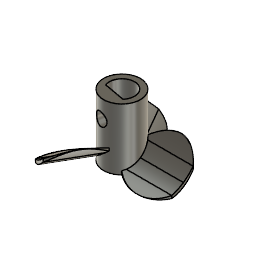
Drill_head_ship_screw (Autodesk Fusion 360 design; units mm, degrees)
Autodesk Fusion 360 part; units mm, degrees
note: some values were not read from the file. Chosen so that the rebuilt part matches the saved one: a direction; which face or edge a step refers to. Set by a fixed rule: which sketch regions a step uses.
sketch "Skizze1" plane through (0, 0, 0) normal (0, 0, 1) x (1, 0, 0)
  circle A0 centre (0, 0) radius 20
  dimension "d1" = 40
  constraint coincident A0.centre origin
  measures "d1" diameter of A0
extrude "Extrusion1" add sketch "Skizze1" along normal blind 10 makes body 1
sketch "Skizze2" plane through (0, 0, 10) normal (0, 0, 1) x (-1, 0, 0)
  circle A0 centre (0, 0) radius 20
  spline S0 degree 5 poles (-19.6944, -3.4827) (-19.4886, -3.7223) (-19.0692, -4.1829) (-18.4174, -4.8178) (-17.5023, -5.5517) (-16.2812, -6.2762) (-14.9841, -6.8018) (-13.6162, -7.1226) (-12.1897, -7.2366) (-10.7248, -7.1467) (-9.2455, -6.859) (-7.7765, -6.381) (-6.3398, -5.7215) (-4.9513, -4.8904) (-3.6191, -3.8981) (-2.3472, -2.7537) (-1.3783, -1.7223) (-0.6787, -0.8855) (-0.2242, -0.2998) (0, 0) knots 0 0 0 0 0 0 0.066667 0.133333 0.2 0.266667 0.333333 0.4 0.466667 0.533333 0.6 0.666667 0.733333 0.8 0.866667 0.933333 1 1 1 1 1 1
  line L0 (0, 0) -> (-20, 0) construction
  spline S1 degree 5 poles (-19.6944, 3.4827) (-19.4886, 3.7223) (-19.0692, 4.1829) (-18.4174, 4.8178) (-17.5023, 5.5517) (-16.2812, 6.2762) (-14.9841, 6.8018) (-13.6162, 7.1226) (-12.1897, 7.2366) (-10.7248, 7.1467) (-9.2455, 6.859) (-7.7765, 6.381) (-6.3398, 5.7215) (-4.9513, 4.8904) (-3.6191, 3.8981) (-2.3472, 2.7537) (-1.3783, 1.7223) (-0.6787, 0.8855) (-0.2242, 0.2998) (0, 0) knots 0 0 0 0 0 0 0.066667 0.133333 0.2 0.266667 0.333333 0.4 0.466667 0.533333 0.6 0.666667 0.733333 0.8 0.866667 0.933333 1 1 1 1 1 1
  line L1 (-21.3276, -1.5819) -> (-18.0612, -5.3835)
  line L2 (-1.5119, -2.0215) -> (1.5119, 2.0215)
  line L3 (-21.3276, 1.5819) -> (-18.0612, 5.3835)
  line L4 (-1.5119, 2.0215) -> (1.5119, -2.0215)
  point P0 (-14, -7)
  point P1 (-7, -6)
  point P2 (-14, 7)
  point P3 (-7, 6)
  constraint coincident A0 S0.start
  constraint coincident A0.centre S0.end
  constraint coincident A0 L0.end
  constraint horizontal L0
  constraint midpoint S0.start L1
  constraint midpoint A0.centre L2
  constraint symmetric S0.start L0 S1.start
  constraint symmetric P0 L0 P2
  constraint symmetric P1 L0 P3
  constraint symmetric A0.centre L0 S0.end
  constraint symmetric L0 L1.start L3.start
  constraint symmetric L0 L1.end L3.end
  constraint symmetric L0 L2.start L4.start
  constraint symmetric L0 L2.end L4.end
extrude "Extrusion2" cut sketch "Skizze2" against normal blind 38 contours A0 S0 S1 picked at (11.5447, -6.597) bodies 1
ref_plane "Arbeitsebene1" through (20, 0, 7.0602) normal (1, 0, 0) x (0, -1, 0)
sketch "Skizze3" plane through (20, 0, 0) normal (1, 0, 0) x (0, 1, 0)
  line L0 (0, 0) -> (-7.1861, 0)
  line L1 (-3.4827, 0) -> (-3.4827, 10)
  line L2 (0, 10) -> (-7.186, 10)
  line L3 (0, 10) -> (0, 0)
  line L4 (0, 0) -> (7.186, 0)
  line L5 (0, 0) -> (0, 10)
  line L6 (0, 10) -> (7.186, 10)
  line L7 (3.4827, 10) -> (3.4827, 0)
  line L8 (-3.4827, 10) -> (-3.4827, 0)
  line L9 (3.4827, 0) -> (-3.4827, 0)
  line L10 (3.4827, 0) -> (3.4827, 10)
  line L11 (3.4827, 10) -> (-3.4827, 10)
  spline S0 degree 5 poles (-7.1861, 0) (-6.8583, 0.0244) (-6.2065, 0.089) (-5.2397, 0.2335) (-3.9728, 0.523) (-2.4286, 1.0564) (-0.9268, 1.7751) (0.5297, 2.691) (1.9406, 3.8055) (3.309, 5.1055) (4.6386, 6.5747) (5.674, 7.8733) (6.4357, 8.9119) (6.937, 9.6326) (7.186, 10) knots 0 0 0 0 0 0 0.1 0.2 0.3 0.4 0.5 0.6 0.7 0.8 0.9 1 1 1 1 1 1
  spline S1 degree 5 poles (-7.1861, 0) (-6.8771, 0.1103) (-6.2612, 0.339) (-5.343, 0.7058) (-4.1304, 1.2436) (-2.6353, 2.0023) (-1.1628, 2.8546) (0.2858, 3.8075) (1.7096, 4.8631) (3.1102, 6.016) (4.4894, 7.2581) (5.5771, 8.3169) (6.3847, 9.1453) (6.9195, 9.7126) (7.186, 10) knots 0 0 0 0 0 0 0.1 0.2 0.3 0.4 0.5 0.6 0.7 0.8 0.9 1 1 1 1 1 1
  point P0 (0, 2.3885)
  point P1 (0, 3.6399)
  constraint coincident L0.end S0.start
  constraint coincident L5 P0
  constraint coincident L6.end S0.end
  constraint coincident L3 P1
extrude "Extrusion3" cut sketch "Skizze3" against normal blind 24 contours L1 L3 L5 L8 S0 S1 | L3 L5 L7 L10 S0 S1 | L1 L8 S0 S1 | L7 L10 S0 S1 keep common part bodies 1
pattern_circular "C-Anordnung1" count 3 over 360 about axis through (0, 0, 1.75) along (0, 0, 1) of bodies 1 makes body 2 at (-7.7524, 7.7486, 4.6885) makes body 3 at (-2.8343, -10.588, 4.6885)
sketch "Skizze4" plane through (0, 0, 0) normal (1, 0, 0) x (0, 1, 0)
sketch "Skizze5" plane through (0, 0, 0) normal (0, 0, 1) x (1, 0, 0)
  circle A0 centre (0, 0) radius 6
  dimension "d11" = 12
  constraint coincident A0.centre origin
  measures "d11" diameter of A0
extrude "Extrusion4" add sketch "Skizze5" along normal blind 20 bodies 1 2 3
sketch "Skizze6" plane through (0, 0, 20) normal (0, 0, 1) x (-1, 0, 0)
  circle A0 centre (0, 0) radius 6
  circle A1 centre (0, 0) radius 4.1
  line L0 (3.8279, 1.4687) -> (-3.0572, 2.732)
  dimension "d16" = 8.2
  dimension "d17" = 7
  constraint concentric A0 A1
  constraint coincident A1 L0.start
  constraint coincident A1 L0.end
  measures "d16" diameter of A1
  measures "d17" distance of L0.start L0.end
extrude "Extrusion6" cut sketch "Skizze6" against normal blind 15 contours A1 L0 picked at (-0.421, -1.6975) bodies 1
ref_plane "Arbeitsebene2" through (-1.0828, -5.9015, 12.5) normal (0.180462, 0.983582, 0) x (0.983582, -0.180462, 0)
sketch "Skizze7" plane through (-1.0828, -5.9015, 0) normal (0.180462, 0.983582, 0) x (0.983582, -0.180462, 0)
  line L0 (-6, -20) -> (6, -20)
  spline S0 degree 3 poles (3.344, -7.1033) (3.6411, -6.872) (3.9199, -6.6249) (4.177, -6.3676) knots -0.132297 -0.132297 -0.132297 -0.132297 0 0 0 0
  line L1 (4.177, -6.3676) -> (18.7426, -6.3676)
  spline S1 degree 3 poles (18.7426, -6.3676) (17.9015, -7.0909) (16.9507, -7.8261) (14.9822, -8.9816) (13.9813, -9.4351) (12.2614, -9.8708) (11.6241, -9.9652) (10.8516, -9.9974) (10.7237, -10) (10.5963, -10) knots -2.032084 -2.032084 -2.032084 -2.032084 -1.639025 -1.639025 -1.298776 -1.298776 -1.101787 -1.101787 -1.062478 -1.062478 -1.062478 -1.062478
  spline S2 degree 3 poles (10.5963, -10) (10.1221, -10) (9.6562, -9.9635) (8.2852, -9.7579) (7.4291, -9.4951) (5.3831, -8.6191) (4.2877, -7.883) (3.344, -7.1033) knots -1.062478 -1.062478 -1.062478 -1.062478 -0.916121 -0.916121 -0.621872 -0.621872 -0.147457 -0.147457 -0.147457 -0.147457
  line L2 (0, -20) -> (0, -14)
  circle A0 centre (0, -14) radius 2.1
  dimension "d21" = 4.2
  constraint midpoint L0 L2.start
  constraint perpendicular L0 L2
  constraint coincident L2.end A0.centre
  measures "d21" diameter of A0
extrude "Extrusion7" cut sketch "Skizze7" along normal blind 3.501 contours A0 bodies 1
extrude "Extrusion8" cut 1 faces at (-0.5906, -2.4324, 14.5906) along direction (0.180462, 0.983582, 0) blind 0.364 on bodies 1 bodies 1
extrude "Extrusion9" [suppressed]
sketch "Skizze8" plane through (0, 0, 30) normal (0, 0, 1) x (-1, 0, 0)
  arc A0 (-3.0572, 2.732) -> (3.8279, 1.4687) centre (0, 0) ccw
  line L0 (-3.0572, 2.732) -> (3.8279, 1.4687)
  circle A1 centre (0, 0) radius 6
  circle A2 centre (0, 0) radius 7.5
  dimension "d28" = 15
  constraint concentric A0 A2
  measures "d28" diameter of A2
extrude "Extrusion10" [suppressed]
